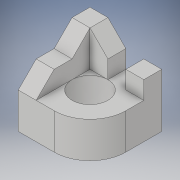
# Autodesk Inventor part: 零件20
Saved by Autodesk Inventor 2019 (Build 230136000, 136)
## iProperties
Created: 2020-09-18
Part Number: 零件20
Material: 一般
Document SubType Name: Modeling
Designer: jay
Density: 1 g/cm^3
Appearance: 預設
Author: jay
Autodesk Inventor part; units mm, degrees
ref_plane "YZ Plane" through (0, 0, 0) normal (1, 0, 0) x (0, 1, 0)
ref_plane "XZ Plane" through (0, 0, 0) normal (0, 1, 0) x (-1, 0, 0)
ref_plane "XY Plane" through (0, 0, 0) normal (0, 0, 1) x (1, 0, 0)
sketch "草圖1" plane through (0, 0, 0) normal (0, 0, 1) x (1, 0, 0)
  line L0 (0, 0) -> (40, 0)
  line L1 (40, 0) -> (40, 40)
  line L2 (40, 40) -> (0, 40)
  line L3 (0, 40) -> (0, 0)
  dimension "d0" = 40
  dimension "d1" = 40
  constraints: 8 end point, 2 parallel, 1 horizontal, 1 perpendicular
  measures "d0" distance of L1.end L2.end
  measures "d1" distance of L0.end L1.end
extrude "擠出1" add sketch "草圖1" along normal blind 40
fillet "圓角1" radius 20 1 edges at (40, 20, 40)
sketch "草圖2" plane through (0, 40, 0) normal (0, 1, 0) x (1, 0, 0)
  arc A0 (20, -40) -> (40, -20) centre (20, -20) ccw projected
  point P0 (0, 0)
  constraints: 1 coincident
hole "孔1" at (20, 40, 20) direction (0, -1, 0) diameter 20 end through all
sketch "草圖3" plane through (0, 40, 0) normal (0, 1, 0) x (1, 0, 0)
  line L0 (0, 0) -> (40, 0) projected
  line L1 (20, 0) -> (30, 0)
  line L2 (30, 0) -> (30, -10)
  line L3 (30, -10) -> (40, -10)
  line L4 (40, 0) -> (40, -20) construction
  circle A0 centre (20, -20) radius 10 construction
  arc A1 (20, -40) -> (40, -20) centre (20, -20) ccw construction
  line L5 (0, -40) -> (20, -40) construction
  line L6 (0, 0) -> (0, -40) projected
  line L7 (0, 0) -> (40, 0) projected
  line L8 (40, 0) -> (40, -20) projected
  line L9 (10, -10) -> (10, -40)
  line L10 (10, -40) -> (40, -40)
  line L11 (40, -40) -> (40, -10)
  line L12 (10, -10) -> (20, -10)
  line L13 (20, -10) -> (20, 0)
  dimension "d12" = 10
  dimension "d13" = 30
  constraints: 16 end point, 5 perpendicular, 3 midpoint, 2 horizontal, 2 vertical, 1 collinear, 1 point on line
  measures "d12" distance of L1.end L2.end
  measures "d13" distance of L9.end L10.end
extrude "擠出2" cut sketch "草圖3" against normal blind 20 contours L0 L2 L3 L8 L11 L10 L9 L12 L13
sketch "草圖4" plane through (10, 40, 10) normal (0, 0, 1) x (1, 0, 0)
  line L0 (0, 0) -> (10, 0) projected
  line L1 (0, 0) -> (0, -20) projected
  line L2 (0, -20) -> (10, -20) projected
  line L3 (10, 0) -> (10, -20) construction
  line L4 (0, 0) -> (10, -10)
  line L5 (10, -10) -> (30, -10)
  line L6 (30, -10) -> (30, 0)
  line L7 (0, 0) -> (10, 0) projected
  line L8 (30, 0) -> (0, 0)
  line L9 (30, 0) -> (30, -20) projected
  point P0 (-10, -40)
  dimension "d16" = 10
  constraints: 8 end point, 2 perpendicular, 1 collinear, 1 horizontal, 1 midpoint
  measures "d16" distance between parallel lines of L5 L8
extrude "擠出3" cut sketch "草圖4" against normal blind 20
sketch "草圖5" plane through (10, 20, 40) normal (1, 0, 0) x (0, 0, -1)
  line L0 (0, 20) -> (30, 20) projected
  line L1 (0, 0) -> (0, 20) projected
  line L2 (0, 0) -> (20, 0) projected
  line L3 (20, 0) -> (30, 0) projected
  line L4 (30, 20) -> (30, 0) projected
  line L5 (30, 20) -> (20, 10)
  line L6 (20, 10) -> (10, 10)
  line L7 (10, 10) -> (0, 0)
  line L8 (0, 20) -> (0, -20) projected
  line L9 (0, 0) -> (0, 20)
  line L10 (0, 20) -> (30, 20)
  point P0 (40, -20)
  dimension "d19" = 10
  dimension "d20" = 10
  dimension "d21" = 10
  constraints: 10 end point, 1 collinear, 1 horizontal, 1 perpendicular
  measures "d19" distance from line of L0 L5.end
  measures "d20" distance from line of L4 L5.end
  measures "d21" distance from line of L1 L6.end
extrude "擠出4" cut sketch "草圖5" against normal blind 20 contours L0 L5 L6 L7 L1
